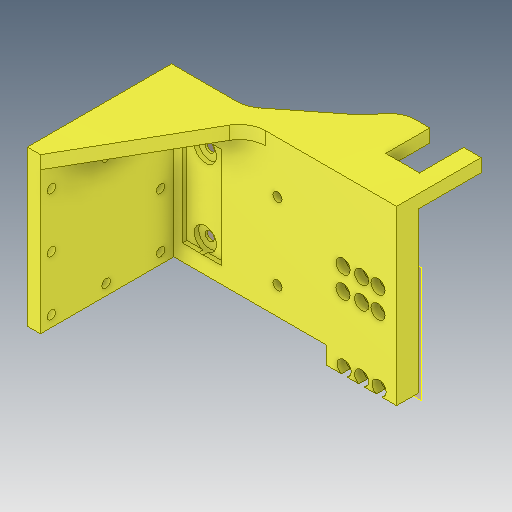
# Autodesk Inventor part: cellSTORM_Lasermount_v0
Saved by Autodesk Inventor 2019 (Build 230136000, 136)
## iProperties
Created: 2019-10-29
Part Number: cellSTORM_Lasermount_v0
Material: Generic
Document SubType Name: Modeling
Designer: diederichbenedict
Density: 1 g/cm^3
Appearance: Smooth - Yellow
Author: diederichbenedict
Autodesk Inventor part; units mm, degrees
ref_plane "YZ Plane" through (0, 0, 0) normal (1, 0, 0) x (0, 1, 0)
ref_plane "XZ Plane" through (0, 0, 0) normal (0, 1, 0) x (-1, 0, 0)
ref_plane "Work Plane1" through (0, 0, 0) normal (0, 0, 1) x (1, 0, 0)
sketch "Sketch1" plane through (0, 0, 0) normal (0, 0, 1) x (1, 0, 0)
  circle A0 centre (23.5, 33) radius 1 construction
  circle A1 centre (23.5, 43) radius 1 construction
  circle A2 centre (24, 3) radius 1 construction
  circle A3 centre (8, 3) radius 1 construction
  circle A4 centre (16, 33) radius 1 construction
  circle A5 centre (16, 43) radius 1 construction
  circle A6 centre (7.5, 43) radius 1 construction
  circle A7 centre (7.5, 33) radius 1.0474 construction
  circle A8 centre (16, 3) radius 1 construction
  line L0 (32, 0) -> (0, 0) construction
  line L1 (32, 0) -> (32, 48) construction
  line L2 (0, 48) -> (32, 48) construction
  line L3 (0, 0) -> (0, 48) construction
  line L4 (7.5277, 79) -> (26, 79) construction
  line L5 (26, 78) -> (7.5277, 78) construction
  line L6 (32, 0) -> (0, 0)
  line L7 (0, 0) -> (0, 79)
  line L8 (0, 79) -> (32, 79)
  line L9 (32, 79) -> (32, 0)
  constraints: 8 end point, 2 parallel, 1 horizontal, 1 perpendicular
ref_plane "Work Plane2" through (-70, 8, 5) normal (0, 0, 1) x (1, 0, 0)
extrude "Extrusion1" add sketch "Sketch1" along normal up to surface (5 mm away)
ref_plane "Work Plane3" through (-40, 38, 5) normal (0, 0, 1) x (0, 1, 0)
sketch "Sketch2" plane through (-40, 38, 5) normal (0, 0, 1) x (0, 1, 0)
  line L0 (28, 30) -> (30, 28) construction
  line L1 (28, 30) -> (-28, 30) construction
  line L2 (-30, 28) -> (-28, 30) construction
  line L3 (-30, 28) -> (-30, -28) construction
  line L4 (-28, -30) -> (-30, -28) construction
  line L5 (-28, -30) -> (28, -30) construction
  line L6 (30, -28) -> (28, -30) construction
  line L7 (30, -28) -> (30, 28) construction
  circle A0 centre (-17.5, -17.5) radius 1.95 construction
  circle A1 centre (17.5, 17.5) radius 1.95 construction
  circle A2 centre (17.5, -17.5) radius 1.95 construction
  circle A3 centre (-17.5, 17.5) radius 1.95 construction
  circle A4 centre (0, 0) radius 7.5 construction
  line L8 (-38, -40) -> (41, -40) construction
  line L9 (-38, -72) -> (-38, -40) construction
  line L10 (41, -72) -> (-38, -72) construction
  line L11 (41, -40) -> (41, -72) construction
  line L12 (41, -40) -> (-30, -40)
  line L13 (-30, -40) -> (-30, 30)
  line L14 (-30, 30) -> (41, 30)
  line L15 (41, 30) -> (41, -40)
  line L16 (41, -72) -> (-38, -72) projected
  line L17 (41, -40) -> (-38, -40)
  line L18 (-38, -40) -> (-38, -72)
  line L19 (-38, -72) -> (41, -72)
  line L20 (41, -72) -> (41, -40)
  point P0 (-38, -40)
  point P1 (41, -50.5)
  constraints: 16 end point, 4 parallel, 2 horizontal, 2 perpendicular, 1 point on line, 1 other
extrude "Extrusion2" add sketch "Sketch2" along normal blind 5
sketch "Sketch3" plane through (-40, 38, 10) normal (0, 0, 1) x (1, 0, 0)
  line L0 (40, -30) -> (40, -38) projected
  line L1 (40, -38) -> (72, -38) projected
  line L2 (72, -38) -> (72, 41) projected
  line L3 (72, 41) -> (-30, 41) projected
  line L4 (-30, 41) -> (-30, -30) projected
  line L5 (-30, -30) -> (40, -30) projected
  circle A0 centre (48, -35) radius 1 projected
  circle A1 centre (64, -35) radius 1 projected
  circle A2 centre (63.5, 5) radius 1 projected
  circle A3 centre (63.5, -5) radius 1 projected
  circle A4 centre (47.5, -5) radius 1.0474 projected
  circle A5 centre (47.5, 5) radius 1 projected
  arc A6 (64.5499, 87.15) -> (61.0499, 90.65) centre (61.0499, 87.15) ccw projected
  line L6 (2.1699, 90.65) -> (61.0499, 90.65) projected
  arc A7 (2.1699, 90.65) -> (-1.3301, 87.15) centre (2.1699, 87.15) ccw projected
  line L7 (-1.3301, -52.85) -> (-1.3301, 87.15) projected
  arc A8 (-1.3301, -52.85) -> (2.1699, -56.35) centre (2.1699, -52.85) ccw projected
  line L8 (61.0499, -56.35) -> (2.1699, -56.35) projected
  arc A9 (61.0499, -56.35) -> (64.5499, -52.85) centre (61.0499, -52.85) ccw projected
  line L9 (64.5499, 87.15) -> (64.5499, -52.85) projected
  circle A10 centre (56, 5) radius 1 projected
  circle A11 centre (56, -5) radius 1 projected
  circle A12 centre (56, -35) radius 1 projected
  point P0 (40, -38)
hole "Hole1" at (7.5, 43, 10) at (16, 43, 10) at (23.5, 43, 10) at (23.5, 33, 10) at (16, 33, 10) at (7.5, 33, 10) at (8, 3, 10) at (16, 3, 10) at (24, 3, 10) direction (0, 0, -1) diameter 3.6 depth 12 tip angle 118 counterbore diameter 6.5 counterbore depth 4
sketch "Sketch4" plane through (-40, 38, 10) normal (0, 0, 1) x (1, 0, 0)
  line L0 (20, -20) -> (-20, -20) projected
  circle A0 centre (-17.5, -17.5) radius 1.95 projected
  circle A1 centre (17.5, -17.5) radius 1.95 projected
  circle A2 centre (17.5, 17.5) radius 1.95 projected
  circle A3 centre (-17.5, 17.5) radius 1.95 projected
  circle A4 centre (-17.5, 17.5) radius 2.1
  point P0 (40, -38)
  dimension "d11" = 4.2
  constraints: 1 centre point, 1 coincident
  measures "d11" diameter of A4
hole "Hole2" at (-57.5, 55.5, 10) at (-22.5, 55.5, 10) at (-22.5, 20.5, 10) at (-57.5, 20.5, 10) direction (0, 0, -1) diameter 4.2 depth 12 tip angle 118
sketch "Sketch5" plane through (0, 79, 0) normal (0, 1, 0) x (1, 0, 0)
  arc A0 (0.1445, 27.7) -> (-0.8555, 28.7) centre (-0.8555, 27.7) ccw construction
  line L0 (-0.8555, 28.7) -> (-4, 28.7) construction
  line L1 (-4, 28.7) -> (-4, 3) construction
  line L2 (-4, 3) -> (5.5277, 3) construction
  arc A1 (5.5277, 3) -> (6.5277, 4) centre (5.5277, 4) ccw construction
  line L3 (6.5277, 4) -> (6.5277, 5.8624) construction
  arc A2 (7.5277, 6.8624) -> (6.5277, 5.8624) centre (7.5277, 5.8624) ccw construction
  line L4 (7.5277, 6.8624) -> (26, 6.8624) construction
  line L5 (26, 6.8624) -> (26, 18.397) construction
  arc A3 (27, 19.397) -> (26, 18.397) centre (27, 18.397) ccw construction
  line L6 (27, 19.397) -> (28, 19.397) construction
  arc A4 (28, 19.397) -> (29, 20.397) centre (28, 20.397) ccw construction
  line L7 (29, 20.397) -> (29, 22.9624) construction
  arc A5 (29, 22.9624) -> (28, 23.9624) centre (28, 22.9624) ccw construction
  line L8 (28, 23.9624) -> (1.1445, 23.9624) construction
  arc A6 (0.1445, 24.9624) -> (1.1445, 23.9624) centre (1.1445, 24.9624) ccw construction
  line L9 (0.1445, 24.9624) -> (0.1445, 27.7) construction
  line L10 (8.5, 22) -> (24, 22) construction
  line L11 (24, 22) -> (24, 8.5) construction
  line L12 (24, 8.5) -> (8.5, 8.5) construction
  line L13 (8.5, 8.5) -> (8.5, 22) construction
  circle A7 centre (-1.5, 26) radius 1 construction
  circle A8 centre (5, 5.5) radius 1 construction
  circle A9 centre (26.5, 21) radius 1 construction
  line L14 (32, 0) -> (32, -10) construction
  line L15 (0, 0) -> (32, 0) construction
  line L16 (0, 0) -> (0, -5) construction
  line L17 (0, -5) -> (-70, -5) construction
  line L18 (-70, -5) -> (-70, -10) construction
  line L19 (32, -10) -> (-70, -10) construction
  line L20 (32, 0) -> (-4, 0)
  line L21 (-4, 0) -> (-4, 28.7)
  line L22 (-4, 28.7) -> (32, 28.7)
  line L23 (32, 28.7) -> (32, 0)
  line L24 (-4, 0) -> (0, 0)
  line L25 (0, 0) -> (0, -5)
  line L26 (0, -5) -> (-4, -5)
  line L27 (-4, -5) -> (-4, 0)
  line L28 (8.5, 28.7) -> (24, 28.7)
  line L29 (24, 28.7) -> (24, 8.5)
  line L30 (24, 8.5) -> (8.5, 8.5)
  line L31 (8.5, 8.5) -> (8.5, 28.7)
  circle A10 centre (5, 5.5) radius 0.75
  circle A11 centre (-1.5, 26) radius 0.75
  circle A12 centre (26.5, 21) radius 0.75
  point P0 (0, 0)
  dimension "d19" = 1.5
  dimension "d20" = 1.5
  dimension "d21" = 1.5
  constraints: 24 end point, 6 parallel, 3 centre point, 3 coincident, 3 horizontal, 3 perpendicular, 1 point on line
  measures "d19" diameter of A10
  measures "d20" diameter of A11
  measures "d21" diameter of A12
extrude "Extrusion3" add sketch "Sketch5" against normal blind 6 contours L20 L21 L22 L31 L30 L29 L23 | L25 L26 L27 L20
sketch "Sketch6" plane through (-70, 8, 5) normal (-1, 0, 0) x (0, 0, 1)
  circle A0 centre (61, 30) radius 1.95 projected
  circle A1 centre (36, 55) radius 1.95 projected
  circle A2 centre (11, 55) radius 1.95 projected
  circle A3 centre (61, 5) radius 1.95 projected
  circle A4 centre (11, 5) radius 1.95 projected
  circle A5 centre (61, 55) radius 1.95 projected
  circle A6 centre (36, 5) radius 1.95 projected
  circle A7 centre (11, 30) radius 1.95 projected
  line L0 (66, 58) -> (64, 60) projected
  line L1 (64, 60) -> (8, 60) projected
  line L2 (8, 60) -> (6, 58) projected
  line L3 (6, 58) -> (6, 2) projected
  line L4 (6, 2) -> (8, 0) projected
  line L5 (8, 0) -> (64, 0) projected
  line L6 (64, 0) -> (66, 2) projected
  line L7 (66, 2) -> (66, 58) projected
  line L8 (0, 71) -> (0, 0) projected
  line L9 (0, 0) -> (5, 0) projected
  line L10 (5, 71) -> (5, 0) projected
  line L11 (0, 71) -> (5, 71) projected
  line L12 (66, 0) -> (0, 0)
  line L13 (0, 0) -> (0, 71)
  line L14 (0, 71) -> (66, 71)
  line L15 (66, 71) -> (66, 0)
  point P0 (-5, -8)
  constraints: 8 end point, 2 parallel, 1 horizontal, 1 perpendicular, 1 point on line
extrude "Extrusion4" add sketch "Sketch6" along normal blind 6
sketch "Sketch7" plane through (-4, 79, -28.7) normal (0, 1, 0) x (1, 0, 0)
  circle A0 centre (9, -23.2) radius 0.75 projected
  circle A1 centre (2.5, -2.7) radius 0.75 projected
  circle A2 centre (30.5, -7.7) radius 0.75 projected
  line L0 (36, -38.7) -> (36, 0) projected
  line L1 (36, 0) -> (28, 0) projected
  line L2 (28, 0) -> (28, -20.2) projected
  line L3 (28, -20.2) -> (12.5, -20.2) projected
  line L4 (12.5, -20.2) -> (12.5, 0) projected
  line L5 (12.5, 0) -> (0, 0) projected
  line L6 (0, 0) -> (0, -33.7) projected
  line L7 (0, -33.7) -> (-72, -33.7) projected
  line L8 (-72, -99.7) -> (-72, -33.7) projected
  line L9 (-66, -99.7) -> (-72, -99.7) projected
  line L10 (-66, -99.7) -> (-66, -38.7) projected
  line L11 (36, -38.7) -> (-66, -38.7) projected
  line L12 (-66, -99.7) -> (-72, -99.7) projected
  line L13 (-66, -99.7) -> (-31, -38.7)
  line L14 (-66, -38.7) -> (4, -38.7) projected
  line L15 (0, 0) -> (0, -33.7) projected
  line L16 (0, -33.7) -> (-72, -33.7) projected
  line L17 (-28.1311, -33.7) -> (0, -33.7)
  line L18 (0, -33.7) -> (0, 0)
  line L19 (-37.7992, -33.7) -> (-28.1311, -33.7)
  line L20 (0, -33.7) -> (0, 0) projected
  line L21 (0, 0) -> (-7.7257, -10.1)
  line L22 (-7.7257, -10.1) -> (-37.7992, -33.7)
  point P0 (4, -28.7)
  constraints: 12 end point, 2 collinear, 2 midpoint, 2 point on line
extrude "Extrusion5" add sketch "Sketch7" against normal blind 6 contours A0 | A1 | A2 | L11 L10 L9 L8 L7 L6 L5 L4 L3 L2 L1 L0 | L13 L10 L11 | L6 L7 L22 L21
sketch "Sketch8" plane through (-40, 38, 10) normal (0, 0, 1) x (1, 0, 0)
  line L0 (0, 28) -> (-10, 28) construction
  line L1 (0, -28) -> (0, 28) construction
  line L2 (-10, -28) -> (0, -28) construction
  line L3 (-10, -28) -> (-10, 28) construction
  line L4 (-10, -28) -> (-10, 28) construction
  line L5 (-10, -28) -> (-20, -28) construction
  line L6 (-20, 28) -> (-20, -28) construction
  line L7 (-10, 28) -> (-20, 28) construction
  circle A0 centre (-17.5, -17.5) radius 2.1 projected
  circle A1 centre (-17.5, 17.5) radius 2.1 projected
  circle A2 centre (-17.5, -17.5) radius 5.1
  circle A3 centre (-17.5, 17.5) radius 5.1
  point P0 (40, -38)
  dimension "d28" = 3
  dimension "d29" = 3
  constraints: 2 centre point
  measures "d28" radial gap between concentric circles of A0 A2
  measures "d29" radial gap between concentric circles of A1 A3
extrude "Extrusion6" cut sketch "Sketch8" against normal blind 4 contours A1 | A2 | A3
sketch "Sketch9" plane through (-40, 38, 10) normal (0, 0, 1) x (1, 0, 0)
  line L0 (-29.973, -22.5) -> (-7.973, -22.5) construction
  line L1 (-7.973, -22.5) -> (-7.973, 23.5) construction
  line L2 (-7.973, 23.5) -> (-29.973, 23.5) construction
  line L3 (-29.973, 23.5) -> (-29.973, -22.5) construction
  line L4 (-30, -30) -> (40, -30) construction
  line L5 (-7.973, -22.5) -> (-25.973, -22.5)
  line L6 (-25.973, -22.5) -> (-25.973, 23.5)
  line L7 (-25.973, 23.5) -> (-7.973, 23.5)
  line L8 (-7.973, 23.5) -> (-7.973, -22.5)
  point P0 (40, -38)
  dimension "d32" = 22
  dimension "d33" = 46
  dimension "d34" = 7.5
  dimension "d35" = 18
  constraints: 16 end point, 4 parallel, 2 horizontal, 2 perpendicular, 1 point on line
  measures "d32" distance of L2.end L1.end
  measures "d33" distance of L1.end L0.end
  measures "d34" distance between parallel lines of L0 L4
  measures "d35" distance of L6.end L7.end
extrude "Extrusion7" cut sketch "Sketch9" against normal blind 2
fillet "Fillet1" radius 12 4 edges at (-35, 76, 10) (-41.7992, 76, 5) (-11.7257, 76, -18.6) (-4, 76, -28.7)
body "Solid1"
